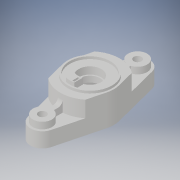
# Autodesk Inventor part: Base
Saved by Autodesk Inventor 2019 (Build 230136000, 136)
## iProperties
Created: 2020-01-30
Part Number: Base
Material: Generic
Document SubType Name: Modeling
Designer: alb16148
Density: 1 g/cm^3
Appearance: Default
Author: alb16148
Autodesk Inventor part; units mm, degrees
ref_plane "YZ Plane" through (0, 0, 0) normal (1, 0, 0) x (0, 1, 0)
ref_plane "XZ Plane" through (0, 0, 0) normal (0, 1, 0) x (-1, 0, 0)
ref_plane "XY Plane" through (0, 0, 0) normal (0, 0, 1) x (1, 0, 0)
sketch "Sketch1" plane through (0, 0, 0) normal (1, 0, 0) x (0, 1, 0)
  line L0 (121, 3) -> (1, 3)
  line L1 (1, 3) -> (1, -3)
  line L2 (1, -3) -> (121, -3)
  line L3 (121, -3) -> (121, 3)
  line L4 (121, 3) -> (1, -3) construction
  line L5 (1, 3) -> (121, -3) construction
  line L6 (10, 8.35) -> (0, 8.35)
  line L7 (0, 8.35) -> (0, 20)
  line L8 (10, 8.35) -> (10, 9.5)
  line L9 (10, 9.5) -> (16, 9.5)
  line L10 (16, 9.5) -> (16, 17)
  line L11 (16, 17) -> (18, 17)
  line L12 (18, 17) -> (18, 18.5)
  line L13 (18, 18.5) -> (16, 18.5)
  line L14 (16, 18.5) -> (16, 20)
  line L15 (16, 20) -> (0, 20)
  line L16 (-36.2, 0) -> (147.2, 0) projected
  line L17 (16, 20) -> (31, 20)
  line L18 (18, 17) -> (31, 17)
  line L19 (75, 9.45) -> (69, 9.45)
  line L20 (69, 9.45) -> (69, 8.35)
  line L21 (69, 8.35) -> (66, 8.35)
  line L22 (75, 9.45) -> (75, 12.45)
  arc A0 (75, 12.45) -> (31, 20) centre (31, -111.9869) ccw
  arc A1 (59.1084, 13.9001) -> (31, 17) centre (31, -111.9869) ccw
  arc A2 (66, 8.35) -> (59.1084, 13.9001) centre (56.9292, 4.1404) ccw
  line L23 (0, 20) -> (-10, 20)
  line L24 (-10, 20) -> (-10, 8.35)
  line L25 (-10, 8.35) -> (0, 8.35)
  line L26 (0, 8.35) -> (0, 20)
  point P0 (0, 0)
  point P1 (61, 0)
  point P2 (61, 0)
  dimension "d0" = 120
  dimension "d1" = 6
  dimension "d5" = 8.35
  dimension "d6" = 9.5
  dimension "d7" = 1.5
  dimension "d8" = 1.5
  dimension "d9" = 20
  dimension "d10" = 6
  dimension "d11" = 2
  dimension "d13" = 10
  dimension "d14" = 1
  dimension "d15" = 6
  dimension "d16" = 3
  dimension "d17" = 9.45
  dimension "d18" = 3
  dimension "d19" = 8.35
  dimension "d20" = 15
  dimension "d21" = 7.5
  dimension "d22" = 75
  dimension "d23" = 10
  dimension "d42" = 10
  dimension "d43" = 8.35
  constraints: 52 end point, 9 perpendicular, 8 horizontal, 6 point on circle, 4 parallel, 3 centre point, 3 midpoint, 3 tangent, 3 vertical, 2 vertical alignment, 1 collinear, 1 concentric, 1 horizontal alignment
  measures "d0" distance of L2.end L1.end
  measures "d1" distance of L1.end L0.end
  measures "d5" distance between parallel lines of L16 L6
  measures "d6" distance between parallel lines of L16 L9
  measures "d7" distance between parallel lines of L15 L13
  measures "d8" distance between parallel lines of L13 L11
  measures "d9" distance between parallel lines of L16 L15
  measures "d10" distance of L8.end L9.end
  measures "d11" distance of L12.end L13.end
  measures "d13" distance of L6.start L6.end
  measures "d14" distance from line of point (0, 0) L1
  measures "d15" distance of L19.start L19.end
  measures "d16" distance of L19.start L22.end
  measures "d17" distance between parallel lines of L16 L19
  measures "d18" distance of L20.end L21.end
  measures "d19" distance between parallel lines of L16 L21
  measures "d20" distance of L14.end L17.end
  measures "d21" distance of L9.end L10.end
  measures "d22" distance between parallel lines of L7 L22
  measures "d23" radius of A2
  measures "d42" distance of L25.end L24.end
  measures "d43" distance between parallel lines of L16 L25
revolve "Revolution1" add sketch "Sketch1" angle 360 about axis through (0, -10, 0) along (0, 1, 0) contours L6 L7 L15 L14 L13 L12 L11 L10 L9 L8 | L25 L24 L23 L7
sketch "Sketch2" plane through (0, 0, 0) normal (0, 1, 0) x (-1, 0, 0)
  circle A0 centre (0, 0) radius 20 projected
  circle A1 centre (0, 40) radius 3.25
  line L0 (28, 0) -> (-28, 0) projected
  line L1 (19.3649, 5) -> (9.6825, 42.5)
  line L2 (-19.3649, 5) -> (-9.6825, 42.5)
  arc A2 (9.6825, 42.5) -> (-9.6825, 42.5) centre (0, 40) ccw
  circle A3 centre (0, 40) radius 8
  arc A4 (15.6149, 19.5237) -> (-15.6149, 19.5237) centre (0, 0) ccw
  line L3 (2, 32.254) -> (2, 24.9199)
  line L4 (-2, 32.254) -> (-2, 24.9199)
  dimension "d25" = 6.5
  dimension "d28" = 10
  dimension "d29" = 16
  dimension "d30" = 5
  dimension "d31" = 40
  dimension "d34" = 4
  constraints: 10 point on circle, 8 end point, 4 centre point, 4 tangent, 3 coincident, 2 point on line, 1 horizontal alignment, 1 parallel, 1 vertical, 1 vertical alignment
  measures "d25" diameter of A1
  measures "d28" radius of A2
  measures "d29" diameter of A3
  measures "d30" radial gap between concentric circles of A0 A4
  measures "d31" distance from line of L0 A1.centre
  measures "d34" distance between parallel lines of L4 L3
extrude "Extrusion1" add sketch "Sketch2" along normal blind 2.5 and the other way blind 10 contours A0 L2 A4 L1 | A4 L3 A3 L4 L2 A2 L1 | A4 L4 A3 L3 | A3 | A1
extrude "Extrusion2" add sketch "Sketch2" along normal up to surface (26 mm away) from surface at -10 contours A0 L2 A4 L1
extrude "Extrusion3" add sketch "Sketch2" along normal blind 8 contours A4 L4 A3 L3 | A3
fillet "Fillet1" radius 4 1 edges at (0, 8, 25)
mirror "Mirror1" about plane through (0, 0, 0) normal (0, 0, 1) of "Extrusion2", "Extrusion3", "Fillet1", "Extrusion1"
sketch "Sketch3" plane through (0, -10, 0) normal (0, -1, 0) x (0, 0, 1)
  line L0 (5, -19.3649) -> (42.5, -9.6825) projected
  circle A0 centre (0, 0) radius 8.35 projected
  arc A1 (-5, -19.3649) -> (5, -19.3649) centre (0, 0) ccw projected
  line L1 (5, -19.3649) -> (42.5, -9.6825) projected
  line L2 (42.5, 9.6825) -> (5, 19.3649) projected
  arc A2 (5, 19.3649) -> (-5, 19.3649) centre (0, 0) ccw projected
  line L3 (-42.5, 9.6825) -> (-5, 19.3649) projected
  line L4 (-5, -19.3649) -> (-42.5, -9.6825) projected
  circle A3 centre (0, 0) radius 8.35 projected
  arc A4 (-5, -19.3649) -> (5, -19.3649) centre (0, 0) ccw projected
  line L5 (5, -19.3649) -> (42.5, -9.6825) projected
  line L6 (42.5, 9.6825) -> (5, 19.3649) projected
  arc A5 (5, 19.3649) -> (-5, 19.3649) centre (0, 0) ccw projected
  line L7 (-42.5, 9.6825) -> (-5, 19.3649) projected
  line L8 (-5, -19.3649) -> (-42.5, -9.6825) projected
  line L9 (20, 10) -> (-20, 10)
  line L10 (-20, 10) -> (-20, -10)
  line L11 (-20, -10) -> (20, -10)
  line L12 (20, -10) -> (20, 10)
  arc A6 (42.5, -9.6825) -> (42.5, 9.6825) centre (40, 0) ccw projected
  arc A7 (-42.5, 9.6825) -> (-42.5, -9.6825) centre (-40, 0) ccw projected
  arc A8 (42.5, -9.6825) -> (42.5, 9.6825) centre (40, 0) ccw projected
  arc A9 (-42.5, 9.6825) -> (-42.5, -9.6825) centre (-40, 0) ccw projected
  point P0 (15.6149, 19.5237)
  dimension "d44" = 0
  dimension "d45" = 0
  dimension "d59" = 40
  dimension "d60" = 10
  dimension "d61" = 10
  constraints: 8 end point, 2 parallel, 1 horizontal, 1 perpendicular, 1 other
  measures "d44" distance edge to line of A1 L12
  measures "d45" distance edge to line of A2 L10
  measures "d59" distance between parallel lines of L10 L12
  measures "d60" distance from line of A0.centre L11
  measures "d61" distance from line of point (0, 0) L9
extrude "Extrusion5" cut sketch "Sketch3" against normal blind 15 contours L12 L11 L10 L9
sketch "Sketch4" plane through (0, -10, 0) normal (0, -1, 0) x (0, 0, 1)
  line L0 (-20, -10) -> (-20, 10) projected
  line L1 (-20, 10) -> (20, 10) projected
  line L2 (20, 10) -> (20, -10) projected
  line L3 (20, -10) -> (-20, -10) projected
  arc A0 (-5, -19.3649) -> (5, -19.3649) centre (0, 0) ccw projected
  line L4 (5, -19.3649) -> (42.5, -9.6825) projected
  line L5 (42.5, 9.6825) -> (5, 19.3649) projected
  arc A1 (5, 19.3649) -> (-5, 19.3649) centre (0, 0) ccw projected
  line L6 (-42.5, 9.6825) -> (-5, 19.3649) projected
  line L7 (-5, -19.3649) -> (-42.5, -9.6825) projected
  line L8 (24, 12.5) -> (-24, 12.5)
  line L9 (-24, 12.5) -> (-24, -12.5)
  line L10 (-24, -12.5) -> (24, -12.5)
  line L11 (24, -12.5) -> (24, 12.5)
  arc A2 (42.5, -9.6825) -> (42.5, 9.6825) centre (40, 0) ccw projected
  arc A3 (-42.5, 9.6825) -> (-42.5, -9.6825) centre (-40, 0) ccw projected
  dimension "d51" = 4
  dimension "d52" = 2.5
  dimension "d53" = 4
  dimension "d54" = 2.5
  constraints: 8 end point, 2 parallel, 1 horizontal, 1 perpendicular
  measures "d51" distance between parallel lines of L11 L2
  measures "d52" distance between parallel lines of L8 L1
  measures "d53" distance between parallel lines of L9 L0
  measures "d54" distance between parallel lines of L10 L3
extrude "Extrusion6" cut sketch "Sketch4" against normal blind 5 contours L11 L10 L9 L8
sketch "Sketch6" plane through (0, 16, 0) normal (0, 1, 0) x (1, 0, 0)
  circle A0 centre (0, 0) radius 17 projected
  circle A1 centre (0, 0) radius 9.5 projected
  line L0 (3.5, -16.6358) -> (3.5, -10.1358)
  line L1 (-3.5, -10.1358) -> (-3.5, -16.6358)
  arc A2 (-3.5, -16.6358) -> (3.5, -16.6358) centre (0, 0) ccw
  arc A3 (-3.5, -9.5123) -> (3.5, -9.5123) centre (0, 0) ccw
  line L2 (-3.5, -9.5123) -> (-3.5, -10.1358)
  line L3 (-12.5, 24) -> (-12.5, -24) projected
  line L4 (3.5, -9.5123) -> (3.5, -10.1358)
  dimension "d69" = 3.5
  dimension "d70" = 3.5
  dimension "d75" = 0
  dimension "d76" = 0
  dimension "d77" = 40.402
  constraints: 8 end point, 4 point on circle, 3 parallel, 2 centre point, 1 point on line, 2 other
  measures "d69" distance from line of point (0, 0) L0
  measures "d70" distance from line of point (0, 0) L1
  measures "d75" distance of point (0, 0) A3.centre
  measures "d76" distance of point (0, 0) A3.centre
extrude "Extrusion7" add sketch "Sketch6" along normal blind 5 contours L1 L2 A3 L4 L0 A0
sketch "Sketch7" plane through (0, 21, 0) normal (0, 1, 0) x (1, 0, 0)
  line L0 (1.2, -16) -> (2.7, -16)
  line L1 (2.7, -16) -> (2.7, -11)
  line L2 (2.7, -11) -> (1.2, -11)
  line L3 (1.2, -11) -> (1.2, -16)
  arc A0 (-3.5, -9.5123) -> (3.5, -9.5123) centre (0, 0) ccw projected
  dimension "d79" = 11
  dimension "d80" = 5
  dimension "d81" = 1.5
  dimension "d82" = 1.2
  constraints: 8 end point, 2 parallel, 1 horizontal, 1 perpendicular
  measures "d79" distance from line of A0.centre L2
  measures "d80" distance between parallel lines of L0 L2
  measures "d81" distance between parallel lines of L1 L3
  measures "d82" distance from line of point (0, 0) L3
extrude "Extrusion8" cut sketch "Sketch7" against normal up to surface (16 mm away)
sketch "Sketch8" plane through (0, 2.5, 0) normal (0, 1, 0) x (1, 0, 0)
  circle A0 centre (0, -40) radius 3.25 projected
  circle A1 centre (0, 40) radius 3.25 projected
  point P0 (0, 0)
extrude "Extrusion9" cut sketch "Sketch8" against normal up to surface (12.5 mm away)
sketch "Sketch9" plane through (-10, 5, -20) normal (0, 0, 1) x (1, 0, 0)
  point P0 (10, -5)
sketch "Sketch10" plane through (-10, 5, -20) normal (0, 0, 1) x (1, 0, 0)
  line L0 (0, -10) -> (0, 0) projected
  line L1 (0, -8) -> (3, -8)
  line L2 (3, -8) -> (3, -3)
  line L3 (3, -3) -> (0, -3)
  line L4 (0, -3) -> (0, -8)
  line L5 (0, -10) -> (20, -10) projected
  line L6 (20, -10) -> (20, 0) projected
  line L7 (20, 0) -> (0, 0) projected
  line L8 (0, -10) -> (0, 0) projected
  point P0 (10, -5)
  point P1 (0, -2.5)
  dimension "d87" = 2
  dimension "d88" = 5
  dimension "d89" = 3
  constraints: 8 end point, 2 parallel, 1 horizontal, 1 perpendicular, 1 point on line
  measures "d87" distance between parallel lines of L1 L5
  measures "d88" distance between parallel lines of L1 L3
  measures "d89" distance between parallel lines of L0 L2
extrude "Extrusion10" cut sketch "Sketch10" against normal blind 30 contours L0 L3 L2 L1
sketch "Sketch11" plane through (0, -5, 0) normal (0, -1, 0) x (1, 0, 0)
  line L0 (-10, -20) -> (10, -20) projected
  line L1 (10, -20) -> (10, 20) projected
  line L2 (-10, -20) -> (10, -20) projected
  line L3 (-10, 20) -> (-10, -20) projected
  line L4 (10, 20) -> (-10, 20) projected
  line L5 (-12.5, -24) -> (-12.5, 24) projected
  line L6 (12.5, -24) -> (-12.5, -24) projected
  line L7 (12.5, 24) -> (12.5, -24) projected
  line L8 (-12.5, 24) -> (12.5, 24) projected
  circle A0 centre (0, -22) radius 1.5
  circle A1 centre (0, 22) radius 1.5
  point P0 (0, 0)
  dimension "d92" = 3
  dimension "d93" = 3
  dimension "d94" = 22
  dimension "d95" = 22
  dimension "d96" = 0
  dimension "d97" = 0
  constraints: 2 centre point
  measures "d92" diameter of A0
  measures "d93" diameter of A1
  measures "d94" distance of A0.centre point (0, 0)
  measures "d95" distance of A1.centre point (0, 0)
  measures "d96" horizontal distance of A0.centre point (0, 0)
  measures "d97" horizontal distance of point (0, 0) A1.centre
extrude "Extrusion11" cut sketch "Sketch11" against normal blind 20 contours A0 | A1
sketch "Sketch12" plane through (-19.3649, -10, -5) normal (-0.9682, 0, -0.25) x (-0.25, 0, 0.9682)
  point P0 (0, 10)
sketch "Sketch14" plane through (0, 5, 0) normal (0, -1, 0) x (1, 0, 0)
  line L0 (2.7, 16) -> (2.7, 11) projected
  line L1 (1.2, 11) -> (1.2, 16) projected
  line L2 (2.7, 11) -> (1.2, 11) projected
  line L3 (1.2, 16) -> (2.7, 16) projected
  line L4 (-8.8, 19) -> (8.7, 19)
  line L5 (8.7, 19) -> (8.7, 10)
  line L6 (8.7, 10) -> (-8.8, 10)
  line L7 (-8.8, 10) -> (-8.8, 19)
  line L8 (-10, 20) -> (10, 20) projected
  point P0 (0, 0)
  dimension "d101" = 1
  dimension "d102" = 6
  dimension "d103" = 10
  dimension "d106" = 1
  constraints: 8 end point, 2 parallel, 1 horizontal, 1 perpendicular
  measures "d101" distance between parallel lines of L6 L2
  measures "d102" distance between parallel lines of L5 L0
  measures "d103" distance between parallel lines of L7 L1
  measures "d106" distance between parallel lines of L8 L4
extrude "Extrusion12" cut sketch "Sketch14" against normal blind 8
equation "\"d61\" = d60"
equation "\"d54\" = d52"
equation "\"d70\" = d69"
equation "\"d95\" = d94"
body "Solid1"
